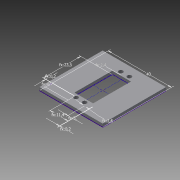
# Autodesk Inventor part: ServoTrace
Saved by Autodesk Inventor 2014 SP1 (Build 180222100, 222)
## iProperties
Created: 2014-01-20
Part Number: ServoTrace
Material: Generic
Document SubType Name: Modeling
Designer: david
Density: 1 g/cm^3
Appearance: Default
Author: david
Autodesk Inventor part; units mm, degrees
ref_plane "YZ Plane" through (0, 0, 0) normal (1, 0, 0) x (0, 1, 0)
ref_plane "XZ Plane" through (0, 0, 0) normal (0, 1, 0) x (-1, 0, 0)
ref_plane "XY Plane" through (0, 0, 0) normal (0, 0, 1) x (1, 0, 0)
sketch "Sketch1" plane through (0, 0, 0) normal (0, 1, 0) x (-1, 0, 0)
  line L0 (-5.7, 11.75) -> (5.7, 11.75) construction
  line L1 (5.7, 11.75) -> (5.7, -11.75) construction
  line L2 (5.7, -11.75) -> (-5.7, -11.75) construction
  line L3 (-5.7, -11.75) -> (-5.7, 11.75) construction
  line L4 (0, 15.7993) -> (0, -16.2311) construction
  line L5 (0, 0) -> (13.9659, 0) construction
  line L6 (-5.7, 16.15) -> (5.7, 16.15) construction
  line L7 (5.7, 16.15) -> (5.7, -16.15) construction
  line L8 (5.7, -16.15) -> (-5.7, -16.15) construction
  line L9 (-5.7, -16.15) -> (-5.7, 16.15) construction
  circle A0 centre (-2.7, 14.15) radius 1.3
  line L10 (0, 0) -> (-13.9659, 0) construction
  circle A1 centre (2.7, 14.15) radius 1.3
  circle A2 centre (-2.7, -14.15) radius 1.3
  circle A3 centre (2.7, -14.15) radius 1.3
  line L11 (-20, 20) -> (20, 20)
  line L12 (20, 20) -> (20, -20)
  line L13 (20, -20) -> (-20, -20)
  line L14 (-20, -20) -> (-20, 20)
  line L15 (0, 0) -> (0, 9.3177) construction
  line L16 (-5.9, 11.95) -> (5.9, 11.95)
  line L17 (5.9, 11.95) -> (5.9, -11.95)
  line L18 (5.9, -11.95) -> (-5.9, -11.95)
  line L19 (-5.9, -11.95) -> (-5.9, 11.95)
  dimension "d1" = 3
  dimension "d2" = 4.4
  dimension "d4" = 23.5
  dimension "d5" = 11.4
  dimension "d6" = 2.6
  dimension "d7" = 40
  dimension "d10" = 0.2
  dimension "d11" = 0.2
  dimension "d14" = 2.4
  constraints: 40 end point, 10 parallel, 6 perpendicular, 4 centre point, 4 horizontal, 4 symmetric about line, 3 collinear, 1 coincident, 10 other
  measures "d1" distance from line of L9 A0.centre
  measures "d2" distance between parallel lines of L6 L0
  measures "d4" distance between parallel lines of L2 L0
  measures "d5" distance between parallel lines of L1 L3
  measures "d6" diameter of A0
  measures "d7" distance of L11.start L11.end
  measures "d10" distance between parallel lines of L0 L16
  measures "d11" distance between parallel lines of L19 L3
  measures "d14" distance from line of L2 A3.centre
extrude "Extrusion2" add sketch "Sketch1" along normal blind 1.9
equation "\"d1\" = ServoEdgeToFixation"
equation "\"d2\" = ServoFixationLength"
equation "\"d4\" = ServoCoreLength"
equation "\"d5\" = ServoCoreWidth"
equation "\"d6\" = ServoScrewDiameterRequired"
equation "\"d10\" = ServoTraceSpacing"
equation "\"d11\" = ServoTraceSpacing"
equation "\"d14\" = ServoCoreToFixation"
equation "\"d12\" = ServoArmThickness"
equation "\"ServoTraceSpacing\" = 0.2"
equation "\"ServoEdgeToFixation\" = 3"
equation "\"ServoFixationLength\" = 4.4"
equation "\"ServoCoreLength\" = 23.5"
equation "\"ServoCoreWidth\" = 11.4"
equation "\"ServoScrewDiameterRequired\" = 2.6"
equation "\"ServoCoreToFixation\" = 2.4"
equation "\"ServoArmThickness\" = 1.9"
body "Solid2"
